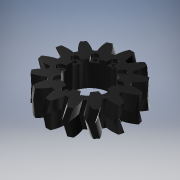
# Autodesk Inventor part: Spur Gear1
Saved by Autodesk Inventor 2017 SP1 (Build 210196100, 196)
## iProperties
Created: 2019-10-27
Part Number: Spur Gear1
Material: ABS Plastic
Document SubType Name: Modeling
Designer: Zach
Categories: <?xml version="1.0" encoding="UTF-16"?> <MemberInstance><Categories><FamilyTemplate><FamilyTemplateParameter ValueType="xs:double" Id="1" ObjectReferenceKey="da_z" ObjectType="kUserParameterObject"/><FamilyTemplateParameter ValueType="xs:double" Id="2" ObjectReferenceKey="da_b" ObjectType="kUserParameterObject"/><FamilyTemplateParameter ValueType="xs:double" Id="3" ObjectReferenceKey="da_beta" ObjectType="kUserParameterObject"/><FamilyTemplateParameter ValueType="xs:double" Id="4" ObjectReferenceKey="da_da" ObjectType="kUserParameterObject"/><FamilyTemplateParameter ValueType="xs:double" Id="5" ObjectReferenceKey="da_aw" ObjectType="kUserParameterObject"/><FamilyTemplateParameter ValueType="xs:string" Id="6" ObjectReferenceKey="EAIAABAAAACIAQAAAAAAAIAAAAAAAAAA" ObjectType="83910656" SubObjectId="SurfaceGeometry"/></FamilyTemplate><ParamToTemplateMap><ParamToTemplate CategoryParameter="//CategoryParameter[@InternalName='046C89C9-8512-4d59-83FE-43B91F4F132A']" TemplateParameter="1"/><ParamToTemplate CategoryParameter="//CategoryParameter[@InternalName='2552DF32-E462-4b46-AEBF-C6C7768E72AC']" TemplateParameter="2"/><ParamToTemplate CategoryParameter="//CategoryParameter[@InternalName='C9EE641D-15FC-4fae-A226-E94C4372FDD7']" TemplateParameter="3"/><ParamToTemplate><ParamToTemplate CategoryParameter="//CategoryParameter[@InternalName='00B6519A-459B-49c7-AD84-2E56D39A5744']" ConstantValue="0.000000"/></ParamToTemplate><ParamToTemplate><ParamToTemplate CategoryParameter="//CategoryParameter[@InternalName='04B31F0E-C7A6-4894-AA32-9629BEFACF47']" ConstantValue="1.000000"/></ParamToTemplate><ParamToTemplate><ParamToTemplate CategoryParameter="//CategoryParameter[@InternalName='43CBEC2E-7847-49e7-A936-2F7889FCB2D9']" ConstantValue="0.250000"/></ParamToTemplate><ParamToTemplate><ParamToTemplate CategoryParameter="//CategoryParameter[@InternalName='B1EFC894-105D-4ebd-86BF-FA20ED196853']" ConstantValue="0.350000"/></ParamToTemplate><ParamToTemplate><ParamToTemplate CategoryParameter="//CategoryParameter[@InternalName='51175063-3D10-4879-93E8-6246FE8B403D']" ConstantValue="2060000000.000000"/></ParamToTemplate><ParamToTemplate><ParamToTemplate CategoryParameter="//CategoryParameter[@InternalName='A3A52E27-4454-46a9-B0BD-C932399B70AF']" ConstantValue="0.300000"/></ParamToTemplate><ParamToTemplate><ParamToTemplate CategoryParameter="//CategoryParameter[@InternalName='91B76062-C214-41d9-B1B9-14D2AB99603D']" ConstantValue="0.300000"/></ParamToTemplate><ParamToTemplate><ParamToTemplate CategoryParameter="//CategoryParameter[@InternalName='374E806E-8B8A-4dda-A9AA-1039D6500AD2']" ConstantValue="3.333333"/></ParamToTemplate><ParamToTemplate><ParamToTemplate CategoryParameter="//CategoryParameter[@InternalName='2D373A89-B862-43d6-8D0B-0CBF12AB9F6C']" ConstantValue="0.392699"/></ParamToTemplate><ParamToTemplate CategoryParameter="//CategoryParameter[@InternalName='37777632-D6A2-4fac-9D53-DB8ACD95C989']" TemplateParameter="4"/><ParamToTemplate CategoryParameter="//CategoryParameter[@InternalName='FD1017F1-B727-4f7e-9707-0F86F1FF9423']" TemplateParameter="5"/><ParamToTemplate><ParamToTemplate CategoryParameter="//CategoryParameter[@InternalName='9E1B4470-B2D3-4ff1-B813-535BB4CDF51A']" ConstantValue="3520000.000000"/></ParamToTemplate><ParamToTemplate><ParamToTemplate CategoryParameter="//CategoryParameter[@InternalName='F8452263-BFF6-458c-9FB1-07C4B99E95CD']" ConstantValue="11400000.000000"/></ParamToTemplate><ParamToTemplate><ParamToTemplate CategoryParameter="//CategoryParameter[@InternalName='3E3BB259-FD49-497f-8171-6EBC954A3479']" ConstantValue="2.000000"/></ParamToTemplate><ParamToTemplate CategoryParameter="//CategoryParameter[@InternalName='27C3BAF2-7550-4e4b-AE2C-0DB134B7D9B7']" TemplateParameter="6"/></ParamToTemplateMap><Category DisplayName="Gear" InternalName="DC85795E-93AB-48d5-8EEE-5A27447B64BD" Mnemonic="Gear"><CategoryParameter DisplayName="z" InternalName="046C89C9-8512-4d59-83FE-43B91F4F132A" Mnemonic="z"/><CategoryParameter DisplayName="b" InternalName="2552DF32-E462-4b46-AEBF-C6C7768E72AC" Mnemonic="b"/><CategoryParameter DisplayName="||b|" InternalName="C9EE641D-15FC-4fae-A226-E94C4372FDD7" Mnemonic="beta"/><CategoryParameter DisplayName="x" InternalName="00B6519A-459B-49c7-AD84-2E56D39A5744" Mnemonic="x"/><CategoryParameter DisplayName="a*" InternalName="04B31F0E-C7A6-4894-AA32-9629BEFACF47" Mnemonic="a"/><CategoryParameter DisplayName="c*" InternalName="43CBEC2E-7847-49e7-A936-2F7889FCB2D9" Mnemonic="c"/><CategoryParameter DisplayName="r|.f|*" InternalName="B1EFC894-105D-4ebd-86BF-FA20ED196853" Mnemonic="rf"/><CategoryParameter DisplayName="E" InternalName="51175063-3D10-4879-93E8-6246FE8B403D" Mnemonic="E"/><CategoryParameter DisplayName="||m|" InternalName="A3A52E27-4454-46a9-B0BD-C932399B70AF" Mnemonic="mi"/><Category DisplayName="SpurGear" InternalName="26C5A22E-A91E-4dfd-A3B3-23CCAFAE1764" Mnemonic="SpurGear"><CategoryParameter DisplayName="m" InternalName="91B76062-C214-41d9-B1B9-14D2AB99603D" Mnemonic="m"/><CategoryParameter DisplayName="P" InternalName="374E806E-8B8A-4dda-A9AA-1039D6500AD2" Mnemonic="PP"/><CategoryParameter DisplayName="||a|" InternalName="2D373A89-B862-43d6-8D0B-0CBF12AB9F6C" Mnemonic="alpha"/><CategoryParameter DisplayName="d|.a|" InternalName="37777632-D6A2-4fac-9D53-DB8ACD95C989" Mnemonic="da"/><CategoryParameter DisplayName="a|.w|" InternalName="FD1017F1-B727-4f7e-9707-0F86F1FF9423" Mnemonic="aw"/><CategoryParameter DisplayName="||s||.Flim|" InternalName="9E1B4470-B2D3-4ff1-B813-535BB4CDF51A" Mnemonic="sFlim"/><CategoryParameter DisplayName="||s||.Hlim|" InternalName="F8452263-BFF6-458c-9FB1-07C4B99E95CD" Mnemonic="sHlim"/><CategoryParameter DisplayName="type" InternalName="3E3BB259-FD49-497f-8171-6EBC954A3479" Mnemonic="type"/><CategoryParameter DisplayName="PitchDiameter" InternalName="27C3BAF2-7550-4e4b-AE2C-0DB134B7D9B7" Mnemonic="IDS_PITCHDIAM"/></Category></Category></Categories></MemberInstance>
Density: 1.06 g/cm^3
Appearance: Smooth - Black
CustomPartVersion: 1
Author: Zach
Autodesk Inventor part; units mm, degrees
ref_plane "YZ Plane" through (0, 0, 0) normal (1, 0, 0) x (0, 1, 0)
ref_plane "XZ Plane" through (0, 0, 0) normal (0, 1, 0) x (-1, 0, 0)
ref_plane "XY Plane" through (0, 0, 0) normal (0, 0, 1) x (1, 0, 0)
sketch "Sketch1" plane through (0, 0, 0) normal (0, 0, 1) x (1, 0, 0)
  circle A0 centre (0, 0) radius 24.740728
  dimension "d0" = 49.48146
  constraints: 1 centre point
  measures "d0" diameter of A0
extrude "Extrusion1" add sketch "Sketch1" along normal blind 7.5
ref_plane "Work Plane2" through (0, 0, 3.75) normal (0, 0, 1) x (1, 0, 0)
sketch "Sketch2" plane through (0, 0, 0) normal (0, 0, -1) x (-1, 0, 0)
  circle A0 centre (0, 0) radius 24.740728
  circle A1 centre (0, 0) radius 21.724138
  dimension "d3" = 43.44828
  constraints: 1 centre point, 1 coincident
  measures "d3" diameter of A1
surface extrude "Pitch Diameter" sketch "Sketch2" against normal through all shown no curves A1
ref_plane "Work Plane8" through (0, 0, 0) normal (0.9749279, 0.2225209, 0) x (0, 0, 1)
ref_plane "Work Plane9" through (0, 0, 0) normal (1, 0, 0) x (0, 1, 0)
spur gear teeth "Spur Gear" teeth 14 pitch diameter 43.4816 tip diameter 49.481455 root diameter 35.9816 face width 7.5 helix angle 15 hand left start plane through (0, 0, 0) normal (0, 0, -1) x (-1, 0, 0)
mirror "Mirror1" about plane through (0, 0, 7.5) normal (0, 0, 1)
sketch "Sketch3" plane through (0, 0, 15) normal (0, 0, 1) x (1, 0, 0)
  circle A0 centre (0, 0) radius 12
  circle A1 centre (0, 14) radius 1.15
  circle A2 centre (-8.228994, 11.326238) radius 1.15
  circle A3 centre (-13.314791, 4.326238) radius 1.15
  circle A4 centre (-13.314791, -4.326238) radius 1.15
  circle A5 centre (-8.228994, -11.326238) radius 1.15
  circle A6 centre (0, -14) radius 1.15
  circle A7 centre (8.228994, -11.326238) radius 1.15
  circle A8 centre (13.314791, -4.326238) radius 1.15
  circle A9 centre (13.314791, 4.326238) radius 1.15
  circle A10 centre (8.228994, 11.326238) radius 1.15
  dimension "d49" = 24
  dimension "d50" = 2.3
  dimension "d51" = 14
  dimension "d54" = 360
  constraints: 11 centre point, 1 coincident, 1 vertical alignment, 21 other
  measures "d49" diameter of A0
  measures "d50" diameter of A1
  measures "d51" distance of point (0, 0) A1.centre
extrude "Extrusion2" cut sketch "Sketch3" against normal through all
sketch "Sketch4" plane through (0, 0, 15) normal (0, 0, 1) x (1, 0, 0)
  circle A0 centre (0, 14) radius 1.15
  circle A1 centre (0, 14) radius 2
  circle A2 centre (-8.228994, 11.326238) radius 2
  circle A3 centre (-13.314791, 4.326238) radius 2
  circle A4 centre (-13.314791, -4.326238) radius 2
  circle A5 centre (-8.228994, -11.326238) radius 2
  circle A6 centre (0, -14) radius 2
  circle A7 centre (8.228994, -11.326238) radius 2
  circle A8 centre (13.314791, -4.326238) radius 2
  circle A9 centre (13.314791, 4.326238) radius 2
  circle A10 centre (8.228994, 11.326238) radius 2
  point P0 (0, 0)
  dimension "d58" = 4
  dimension "d61" = 360
  constraints: 10 centre point, 1 coincident, 21 other
  measures "d58" diameter of A1
extrude "Extrusion3" cut sketch "Sketch4" against normal blind 2 contours A0 | A1 | A2 | A3 | A4 | A5 | A6 | A7 | A8 | A9 | A10
sketch "Sketch5" plane through (0, 0, 15) normal (0, 0, 1) x (1, 0, 0)
  circle A0 centre (0, 14) radius 2
  line L0 (-2, 14) -> (-2, 11.83216)
  line L1 (-2, 11.83216) -> (2, 11.83216)
  line L2 (2, 11.83216) -> (2, 14)
  line L3 (2, 14) -> (-2, 14)
  arc A1 (0, 12) -> (-7.053423, 9.708204) centre (0, 0) ccw
  arc A2 (7.053423, 9.708204) -> (0, 12) centre (0, 0) ccw
  line L4 (-9.847028, 10.150667) -> (-8.572803, 8.396848)
  line L5 (-8.572803, 8.396848) -> (-5.336735, 10.747989)
  line L6 (-5.336735, 10.747989) -> (-6.61096, 12.501808)
  line L7 (-6.61096, 12.501808) -> (-9.847028, 10.150667)
  line L8 (-13.932825, 2.424125) -> (-11.871086, 1.754225)
  line L9 (-11.871086, 1.754225) -> (-10.635018, 5.558451)
  line L10 (-10.635018, 5.558451) -> (-12.696757, 6.228351)
  line L11 (-12.696757, 6.228351) -> (-13.932825, 2.424125)
  line L12 (-12.696757, -6.228351) -> (-10.635018, -5.558451)
  line L13 (-10.635018, -5.558451) -> (-11.871086, -1.754225)
  line L14 (-11.871086, -1.754225) -> (-13.932825, -2.424125)
  line L15 (-13.932825, -2.424125) -> (-12.696757, -6.228351)
  line L16 (-6.61096, -12.501808) -> (-5.336735, -10.747989)
  line L17 (-5.336735, -10.747989) -> (-8.572803, -8.396848)
  line L18 (-8.572803, -8.396848) -> (-9.847028, -10.150667)
  line L19 (-9.847028, -10.150667) -> (-6.61096, -12.501808)
  line L20 (2, -14) -> (2, -11.83216)
  line L21 (2, -11.83216) -> (-2, -11.83216)
  line L22 (-2, -11.83216) -> (-2, -14)
  line L23 (-2, -14) -> (2, -14)
  line L24 (9.847028, -10.150667) -> (8.572803, -8.396848)
  line L25 (8.572803, -8.396848) -> (5.336735, -10.747989)
  line L26 (5.336735, -10.747989) -> (6.61096, -12.501808)
  line L27 (6.61096, -12.501808) -> (9.847028, -10.150667)
  line L28 (13.932825, -2.424125) -> (11.871086, -1.754225)
  line L29 (11.871086, -1.754225) -> (10.635018, -5.558451)
  line L30 (10.635018, -5.558451) -> (12.696757, -6.228351)
  line L31 (12.696757, -6.228351) -> (13.932825, -2.424125)
  line L32 (12.696757, 6.228351) -> (10.635018, 5.558451)
  line L33 (10.635018, 5.558451) -> (11.871086, 1.754225)
  line L34 (11.871086, 1.754225) -> (13.932825, 2.424125)
  line L35 (13.932825, 2.424125) -> (12.696757, 6.228351)
  line L36 (6.61096, 12.501808) -> (5.336735, 10.747989)
  line L37 (5.336735, 10.747989) -> (8.572803, 8.396848)
  line L38 (8.572803, 8.396848) -> (9.847028, 10.150667)
  line L39 (9.847028, 10.150667) -> (6.61096, 12.501808)
  dimension "d67" = 360
  constraints: 80 end point, 4 point on circle, 2 perpendicular, 1 tangent, 1 vertical, 81 other
extrude "Extrusion4" cut sketch "Sketch5" against normal up to surface (2 mm away) from surface at 0
equation "\"d0\" = da_da"
equation "\"d1\" = da_b"
equation "\"d3\" = da_dw"
equation "\"d16\" = da_aw"
equation "\"d43\" = da_aw"
equation "\"d46\" = da_aw"
equation "\"da_da\" = 49.481455"
equation "\"da_b\" = 7.5"
equation "\"da_dw\" = 43.448276"
equation "\"da_aw\" = 45"
body "Solid1"
body "Srf1"
